Autodesk Fusion 360 part; units mm, degrees
(part 2 of 3)
  line L639 (-140.3467, 118.52) -> (-149.3467, 118.52)
  line L640 (-149.3467, 118.52) -> (-149.3467, 112.02)
  line L641 (-140.3467, 112.02) -> (-140.3467, 118.52)
  line L642 (-149.3467, 112.02) -> (-140.3467, 112.02)
  line L643 (-148.7467, 117.92) -> (-148.7467, 112.62)
  line L644 (-140.9467, 117.92) -> (-148.7467, 117.92)
  line L645 (-140.9467, 112.62) -> (-140.9467, 117.92)
  line L646 (-158.6, 112.62) -> (-150.8, 112.62)
  line L647 (-150.2, 118.52) -> (-159.2, 118.52)
  line L648 (-159.2, 118.52) -> (-159.2, 112.02)
  line L649 (-150.2, 112.02) -> (-150.2, 118.52)
  line L650 (-159.2, 112.02) -> (-150.2, 112.02)
  line L651 (-158.6, 117.92) -> (-158.6, 112.62)
  line L652 (-150.8, 117.92) -> (-158.6, 117.92)
  line L653 (-150.8, 112.62) -> (-150.8, 117.92)
  line L654 (-10.8, 102.6) -> (-3, 102.6)
  line L655 (-2.4, 108.5) -> (-11.4, 108.5)
  line L656 (-11.4, 108.5) -> (-11.4, 102)
  line L657 (-2.4, 102) -> (-2.4, 108.5)
  line L658 (-11.4, 102) -> (-2.4, 102)
  line L659 (-10.8, 107.9) -> (-10.8, 102.6)
  line L660 (-3, 107.9) -> (-10.8, 107.9)
  line L661 (-3, 102.6) -> (-3, 107.9)
  line L662 (-20.6533, 102.6) -> (-12.8533, 102.6)
  line L663 (-12.2533, 108.5) -> (-21.2533, 108.5)
  line L664 (-21.2533, 108.5) -> (-21.2533, 102)
  line L665 (-12.2533, 102) -> (-12.2533, 108.5)
  line L666 (-21.2533, 102) -> (-12.2533, 102)
  line L667 (-20.6533, 107.9) -> (-20.6533, 102.6)
  line L668 (-12.8533, 107.9) -> (-20.6533, 107.9)
  line L669 (-12.8533, 102.6) -> (-12.8533, 107.9)
  line L670 (-30.5067, 102.6) -> (-22.7067, 102.6)
  line L671 (-22.1067, 108.5) -> (-31.1067, 108.5)
  line L672 (-31.1067, 108.5) -> (-31.1067, 102)
  line L673 (-22.1067, 102) -> (-22.1067, 108.5)
  line L674 (-31.1067, 102) -> (-22.1067, 102)
  line L675 (-30.5067, 107.9) -> (-30.5067, 102.6)
  line L676 (-22.7067, 107.9) -> (-30.5067, 107.9)
  line L677 (-22.7067, 102.6) -> (-22.7067, 107.9)
  line L678 (-40.36, 102.6) -> (-32.56, 102.6)
  line L679 (-31.96, 108.5) -> (-40.96, 108.5)
  line L680 (-40.96, 108.5) -> (-40.96, 102)
  line L681 (-31.96, 102) -> (-31.96, 108.5)
  line L682 (-40.96, 102) -> (-31.96, 102)
  line L683 (-40.36, 107.9) -> (-40.36, 102.6)
  line L684 (-32.56, 107.9) -> (-40.36, 107.9)
  line L685 (-32.56, 102.6) -> (-32.56, 107.9)
  line L686 (-50.2133, 102.6) -> (-42.4133, 102.6)
  line L687 (-41.8133, 108.5) -> (-50.8133, 108.5)
  line L688 (-50.8133, 108.5) -> (-50.8133, 102)
  line L689 (-41.8133, 102) -> (-41.8133, 108.5)
  line L690 (-50.8133, 102) -> (-41.8133, 102)
  line L691 (-50.2133, 107.9) -> (-50.2133, 102.6)
  line L692 (-42.4133, 107.9) -> (-50.2133, 107.9)
  line L693 (-42.4133, 102.6) -> (-42.4133, 107.9)
  line L694 (-60.0667, 102.6) -> (-52.2667, 102.6)
  line L695 (-51.6667, 108.5) -> (-60.6667, 108.5)
  line L696 (-60.6667, 108.5) -> (-60.6667, 102)
  line L697 (-51.6667, 102) -> (-51.6667, 108.5)
  line L698 (-60.6667, 102) -> (-51.6667, 102)
  line L699 (-60.0667, 107.9) -> (-60.0667, 102.6)
  line L700 (-52.2667, 107.9) -> (-60.0667, 107.9)
  line L701 (-52.2667, 102.6) -> (-52.2667, 107.9)
  line L702 (-69.92, 102.6) -> (-62.12, 102.6)
  line L703 (-61.52, 108.5) -> (-70.52, 108.5)
  line L704 (-70.52, 108.5) -> (-70.52, 102)
  line L705 (-61.52, 102) -> (-61.52, 108.5)
  line L706 (-70.52, 102) -> (-61.52, 102)
  line L707 (-69.92, 107.9) -> (-69.92, 102.6)
  line L708 (-62.12, 107.9) -> (-69.92, 107.9)
  line L709 (-62.12, 102.6) -> (-62.12, 107.9)
  line L710 (-79.7733, 102.6) -> (-71.9733, 102.6)
  line L711 (-71.3733, 108.5) -> (-80.3733, 108.5)
  line L712 (-80.3733, 108.5) -> (-80.3733, 102)
  line L713 (-71.3733, 102) -> (-71.3733, 108.5)
  line L714 (-80.3733, 102) -> (-71.3733, 102)
  line L715 (-79.7733, 107.9) -> (-79.7733, 102.6)
  line L716 (-71.9733, 107.9) -> (-79.7733, 107.9)
  line L717 (-71.9733, 102.6) -> (-71.9733, 107.9)
  line L718 (-89.6267, 102.6) -> (-81.8267, 102.6)
  line L719 (-81.2267, 108.5) -> (-90.2267, 108.5)
  line L720 (-90.2267, 108.5) -> (-90.2267, 102)
  line L721 (-81.2267, 102) -> (-81.2267, 108.5)
  line L722 (-90.2267, 102) -> (-81.2267, 102)
  line L723 (-89.6267, 107.9) -> (-89.6267, 102.6)
  line L724 (-81.8267, 107.9) -> (-89.6267, 107.9)
  line L725 (-81.8267, 102.6) -> (-81.8267, 107.9)
  line L726 (-99.48, 102.6) -> (-91.68, 102.6)
  line L727 (-91.08, 108.5) -> (-100.08, 108.5)
  line L728 (-100.08, 108.5) -> (-100.08, 102)
  line L729 (-91.08, 102) -> (-91.08, 108.5)
  line L730 (-100.08, 102) -> (-91.08, 102)
  line L731 (-99.48, 107.9) -> (-99.48, 102.6)
  line L732 (-91.68, 107.9) -> (-99.48, 107.9)
  line L733 (-91.68, 102.6) -> (-91.68, 107.9)
  line L734 (-109.3333, 102.6) -> (-101.5333, 102.6)
  line L735 (-100.9333, 108.5) -> (-109.9333, 108.5)
  line L736 (-109.9333, 108.5) -> (-109.9333, 102)
  line L737 (-100.9333, 102) -> (-100.9333, 108.5)
  line L738 (-109.9333, 102) -> (-100.9333, 102)
  line L739 (-109.3333, 107.9) -> (-109.3333, 102.6)
  line L740 (-101.5333, 107.9) -> (-109.3333, 107.9)
  line L741 (-101.5333, 102.6) -> (-101.5333, 107.9)
  line L742 (-119.1867, 102.6) -> (-111.3867, 102.6)
  line L743 (-110.7867, 108.5) -> (-119.7867, 108.5)
  line L744 (-119.7867, 108.5) -> (-119.7867, 102)
  line L745 (-110.7867, 102) -> (-110.7867, 108.5)
  line L746 (-119.7867, 102) -> (-110.7867, 102)
  line L747 (-119.1867, 107.9) -> (-119.1867, 102.6)
  line L748 (-111.3867, 107.9) -> (-119.1867, 107.9)
  line L749 (-111.3867, 102.6) -> (-111.3867, 107.9)
  line L750 (-129.04, 102.6) -> (-121.24, 102.6)
  line L751 (-120.64, 108.5) -> (-129.64, 108.5)
  line L752 (-129.64, 108.5) -> (-129.64, 102)
  line L753 (-120.64, 102) -> (-120.64, 108.5)
  line L754 (-129.64, 102) -> (-120.64, 102)
  line L755 (-129.04, 107.9) -> (-129.04, 102.6)
  line L756 (-121.24, 107.9) -> (-129.04, 107.9)
  line L757 (-121.24, 102.6) -> (-121.24, 107.9)
  line L758 (-138.8933, 102.6) -> (-131.0933, 102.6)
  line L759 (-130.4933, 108.5) -> (-139.4933, 108.5)
  line L760 (-139.4933, 108.5) -> (-139.4933, 102)
  line L761 (-130.4933, 102) -> (-130.4933, 108.5)
  line L762 (-139.4933, 102) -> (-130.4933, 102)
  line L763 (-138.8933, 107.9) -> (-138.8933, 102.6)
  line L764 (-131.0933, 107.9) -> (-138.8933, 107.9)
  line L765 (-131.0933, 102.6) -> (-131.0933, 107.9)
  line L766 (-148.7467, 102.6) -> (-140.9467, 102.6)
  line L767 (-140.3467, 108.5) -> (-149.3467, 108.5)
  line L768 (-149.3467, 108.5) -> (-149.3467, 102)
  line L769 (-140.3467, 102) -> (-140.3467, 108.5)
  line L770 (-149.3467, 102) -> (-140.3467, 102)
  line L771 (-148.7467, 107.9) -> (-148.7467, 102.6)
  line L772 (-140.9467, 107.9) -> (-148.7467, 107.9)
  line L773 (-140.9467, 102.6) -> (-140.9467, 107.9)
  line L774 (-158.6, 102.6) -> (-150.8, 102.6)
  line L775 (-150.2, 108.5) -> (-159.2, 108.5)
  line L776 (-159.2, 108.5) -> (-159.2, 102)
  line L777 (-150.2, 102) -> (-150.2, 108.5)
  line L778 (-159.2, 102) -> (-150.2, 102)
  line L779 (-158.6, 107.9) -> (-158.6, 102.6)
  line L780 (-150.8, 107.9) -> (-158.6, 107.9)
  line L781 (-150.8, 102.6) -> (-150.8, 107.9)
  line L782 (-10.8, 92.58) -> (-3, 92.58)
  line L783 (-2.4, 98.48) -> (-11.4, 98.48)
  line L784 (-11.4, 98.48) -> (-11.4, 91.98)
  line L785 (-2.4, 91.98) -> (-2.4, 98.48)
  line L786 (-11.4, 91.98) -> (-2.4, 91.98)
  line L787 (-10.8, 97.88) -> (-10.8, 92.58)
  line L788 (-3, 97.88) -> (-10.8, 97.88)
  line L789 (-3, 92.58) -> (-3, 97.88)
  line L790 (-20.6533, 92.58) -> (-12.8533, 92.58)
  line L791 (-12.2533, 98.48) -> (-21.2533, 98.48)
  line L792 (-21.2533, 98.48) -> (-21.2533, 91.98)
  line L793 (-12.2533, 91.98) -> (-12.2533, 98.48)
  line L794 (-21.2533, 91.98) -> (-12.2533, 91.98)
  line L795 (-20.6533, 97.88) -> (-20.6533, 92.58)
  line L796 (-12.8533, 97.88) -> (-20.6533, 97.88)
  line L797 (-12.8533, 92.58) -> (-12.8533, 97.88)
  line L798 (-30.5067, 92.58) -> (-22.7067, 92.58)
  line L799 (-22.1067, 98.48) -> (-31.1067, 98.48)
  line L800 (-31.1067, 98.48) -> (-31.1067, 91.98)
  line L801 (-22.1067, 91.98) -> (-22.1067, 98.48)
  line L802 (-31.1067, 91.98) -> (-22.1067, 91.98)
  line L803 (-30.5067, 97.88) -> (-30.5067, 92.58)
  line L804 (-22.7067, 97.88) -> (-30.5067, 97.88)
  line L805 (-22.7067, 92.58) -> (-22.7067, 97.88)
  line L806 (-40.36, 92.58) -> (-32.56, 92.58)
  line L807 (-31.96, 98.48) -> (-40.96, 98.48)
  line L808 (-40.96, 98.48) -> (-40.96, 91.98)
  line L809 (-31.96, 91.98) -> (-31.96, 98.48)
  line L810 (-40.96, 91.98) -> (-31.96, 91.98)
  line L811 (-40.36, 97.88) -> (-40.36, 92.58)
  line L812 (-32.56, 97.88) -> (-40.36, 97.88)
  line L813 (-32.56, 92.58) -> (-32.56, 97.88)
  line L814 (-50.2133, 92.58) -> (-42.4133, 92.58)
  line L815 (-41.8133, 98.48) -> (-50.8133, 98.48)
  line L816 (-50.8133, 98.48) -> (-50.8133, 91.98)
  line L817 (-41.8133, 91.98) -> (-41.8133, 98.48)
  line L818 (-50.8133, 91.98) -> (-41.8133, 91.98)
  line L819 (-50.2133, 97.88) -> (-50.2133, 92.58)
  line L820 (-42.4133, 97.88) -> (-50.2133, 97.88)
  line L821 (-42.4133, 92.58) -> (-42.4133, 97.88)
  line L822 (-60.0667, 92.58) -> (-52.2667, 92.58)
  line L823 (-51.6667, 98.48) -> (-60.6667, 98.48)
  line L824 (-60.6667, 98.48) -> (-60.6667, 91.98)
  line L825 (-51.6667, 91.98) -> (-51.6667, 98.48)
  line L826 (-60.6667, 91.98) -> (-51.6667, 91.98)
  line L827 (-60.0667, 97.88) -> (-60.0667, 92.58)
  line L828 (-52.2667, 97.88) -> (-60.0667, 97.88)
  line L829 (-52.2667, 92.58) -> (-52.2667, 97.88)
  line L830 (-69.92, 92.58) -> (-62.12, 92.58)
  line L831 (-61.52, 98.48) -> (-70.52, 98.48)
  line L832 (-70.52, 98.48) -> (-70.52, 91.98)
  line L833 (-61.52, 91.98) -> (-61.52, 98.48)
  line L834 (-70.52, 91.98) -> (-61.52, 91.98)
  line L835 (-69.92, 97.88) -> (-69.92, 92.58)
  line L836 (-62.12, 97.88) -> (-69.92, 97.88)
  line L837 (-62.12, 92.58) -> (-62.12, 97.88)
  line L838 (-79.7733, 92.58) -> (-71.9733, 92.58)
  line L839 (-71.3733, 98.48) -> (-80.3733, 98.48)
  line L840 (-80.3733, 98.48) -> (-80.3733, 91.98)
  line L841 (-71.3733, 91.98) -> (-71.3733, 98.48)
  line L842 (-80.3733, 91.98) -> (-71.3733, 91.98)
  line L843 (-79.7733, 97.88) -> (-79.7733, 92.58)
  line L844 (-71.9733, 97.88) -> (-79.7733, 97.88)
  line L845 (-71.9733, 92.58) -> (-71.9733, 97.88)
  line L846 (-89.6267, 92.58) -> (-81.8267, 92.58)
  line L847 (-81.2267, 98.48) -> (-90.2267, 98.48)
  line L848 (-90.2267, 98.48) -> (-90.2267, 91.98)
  line L849 (-81.2267, 91.98) -> (-81.2267, 98.48)
  line L850 (-90.2267, 91.98) -> (-81.2267, 91.98)
  line L851 (-89.6267, 97.88) -> (-89.6267, 92.58)
  line L852 (-81.8267, 97.88) -> (-89.6267, 97.88)
  line L853 (-81.8267, 92.58) -> (-81.8267, 97.88)
  line L854 (-99.48, 92.58) -> (-91.68, 92.58)
  line L855 (-91.08, 98.48) -> (-100.08, 98.48)
  line L856 (-100.08, 98.48) -> (-100.08, 91.98)
  line L857 (-91.08, 91.98) -> (-91.08, 98.48)
  line L858 (-100.08, 91.98) -> (-91.08, 91.98)
  line L859 (-99.48, 97.88) -> (-99.48, 92.58)
  line L860 (-91.68, 97.88) -> (-99.48, 97.88)
  line L861 (-91.68, 92.58) -> (-91.68, 97.88)
  line L862 (-109.3333, 92.58) -> (-101.5333, 92.58)
  line L863 (-100.9333, 98.48) -> (-109.9333, 98.48)
  line L864 (-109.9333, 98.48) -> (-109.9333, 91.98)
  line L865 (-100.9333, 91.98) -> (-100.9333, 98.48)
  line L866 (-109.9333, 91.98) -> (-100.9333, 91.98)
  line L867 (-109.3333, 97.88) -> (-109.3333, 92.58)
  line L868 (-101.5333, 97.88) -> (-109.3333, 97.88)
  line L869 (-101.5333, 92.58) -> (-101.5333, 97.88)
  line L870 (-119.1867, 92.58) -> (-111.3867, 92.58)
  line L871 (-110.7867, 98.48) -> (-119.7867, 98.48)
  line L872 (-119.7867, 98.48) -> (-119.7867, 91.98)
  line L873 (-110.7867, 91.98) -> (-110.7867, 98.48)
  line L874 (-119.7867, 91.98) -> (-110.7867, 91.98)
  line L875 (-119.1867, 97.88) -> (-119.1867, 92.58)
  line L876 (-111.3867, 97.88) -> (-119.1867, 97.88)
  line L877 (-111.3867, 92.58) -> (-111.3867, 97.88)
  line L878 (-129.04, 92.58) -> (-121.24, 92.58)
  line L879 (-120.64, 98.48) -> (-129.64, 98.48)
  line L880 (-129.64, 98.48) -> (-129.64, 91.98)
  line L881 (-120.64, 91.98) -> (-120.64, 98.48)
  line L882 (-129.64, 91.98) -> (-120.64, 91.98)
  line L883 (-129.04, 97.88) -> (-129.04, 92.58)
  line L884 (-121.24, 97.88) -> (-129.04, 97.88)
  line L885 (-121.24, 92.58) -> (-121.24, 97.88)
  line L886 (-138.8933, 92.58) -> (-131.0933, 92.58)
  line L887 (-130.4933, 98.48) -> (-139.4933, 98.48)
  line L888 (-139.4933, 98.48) -> (-139.4933, 91.98)
  line L889 (-130.4933, 91.98) -> (-130.4933, 98.48)
  line L890 (-139.4933, 91.98) -> (-130.4933, 91.98)
  line L891 (-138.8933, 97.88) -> (-138.8933, 92.58)
  line L892 (-131.0933, 97.88) -> (-138.8933, 97.88)
  line L893 (-131.0933, 92.58) -> (-131.0933, 97.88)
  line L894 (-148.7467, 92.58) -> (-140.9467, 92.58)
  line L895 (-140.3467, 98.48) -> (-149.3467, 98.48)
  line L896 (-149.3467, 98.48) -> (-149.3467, 91.98)
  line L897 (-140.3467, 91.98) -> (-140.3467, 98.48)
  line L898 (-149.3467, 91.98) -> (-140.3467, 91.98)
  line L899 (-148.7467, 97.88) -> (-148.7467, 92.58)
  line L900 (-140.9467, 97.88) -> (-148.7467, 97.88)
  line L901 (-140.9467, 92.58) -> (-140.9467, 97.88)
  line L902 (-158.6, 92.58) -> (-150.8, 92.58)
  line L903 (-150.2, 98.48) -> (-159.2, 98.48)
  line L904 (-159.2, 98.48) -> (-159.2, 91.98)
  line L905 (-150.2, 91.98) -> (-150.2, 98.48)
  line L906 (-159.2, 91.98) -> (-150.2, 91.98)
  line L907 (-158.6, 97.88) -> (-158.6, 92.58)
  line L908 (-150.8, 97.88) -> (-158.6, 97.88)
  line L909 (-150.8, 92.58) -> (-150.8, 97.88)
  line L910 (-10.8, 82.56) -> (-3, 82.56)
  line L911 (-2.4, 88.46) -> (-11.4, 88.46)
  line L912 (-11.4, 88.46) -> (-11.4, 81.96)
  line L913 (-2.4, 81.96) -> (-2.4, 88.46)
  line L914 (-11.4, 81.96) -> (-2.4, 81.96)
  line L915 (-10.8, 87.86) -> (-10.8, 82.56)
  line L916 (-3, 87.86) -> (-10.8, 87.86)
  line L917 (-3, 82.56) -> (-3, 87.86)
  line L918 (-20.6533, 82.56) -> (-12.8533, 82.56)
  line L919 (-12.2533, 88.46) -> (-21.2533, 88.46)
  line L920 (-21.2533, 88.46) -> (-21.2533, 81.96)
  line L921 (-12.2533, 81.96) -> (-12.2533, 88.46)
  line L922 (-21.2533, 81.96) -> (-12.2533, 81.96)
  line L923 (-20.6533, 87.86) -> (-20.6533, 82.56)
  line L924 (-12.8533, 87.86) -> (-20.6533, 87.86)
  line L925 (-12.8533, 82.56) -> (-12.8533, 87.86)
  line L926 (-30.5067, 82.56) -> (-22.7067, 82.56)
  line L927 (-22.1067, 88.46) -> (-31.1067, 88.46)
  line L928 (-31.1067, 88.46) -> (-31.1067, 81.96)
  line L929 (-22.1067, 81.96) -> (-22.1067, 88.46)
  line L930 (-31.1067, 81.96) -> (-22.1067, 81.96)
  line L931 (-30.5067, 87.86) -> (-30.5067, 82.56)
  line L932 (-22.7067, 87.86) -> (-30.5067, 87.86)
  line L933 (-22.7067, 82.56) -> (-22.7067, 87.86)
  line L934 (-40.36, 82.56) -> (-32.56, 82.56)
  line L935 (-31.96, 88.46) -> (-40.96, 88.46)
  line L936 (-40.96, 88.46) -> (-40.96, 81.96)
  line L937 (-31.96, 81.96) -> (-31.96, 88.46)
  line L938 (-40.96, 81.96) -> (-31.96, 81.96)
  line L939 (-40.36, 87.86) -> (-40.36, 82.56)
  line L940 (-32.56, 87.86) -> (-40.36, 87.86)
  line L941 (-32.56, 82.56) -> (-32.56, 87.86)
  line L942 (-50.2133, 82.56) -> (-42.4133, 82.56)
  line L943 (-41.8133, 88.46) -> (-50.8133, 88.46)
  line L944 (-50.8133, 88.46) -> (-50.8133, 81.96)
  line L945 (-41.8133, 81.96) -> (-41.8133, 88.46)
  line L946 (-50.8133, 81.96) -> (-41.8133, 81.96)
  line L947 (-50.2133, 87.86) -> (-50.2133, 82.56)
  line L948 (-42.4133, 87.86) -> (-50.2133, 87.86)
  line L949 (-42.4133, 82.56) -> (-42.4133, 87.86)
  line L950 (-60.0667, 82.56) -> (-52.2667, 82.56)
  line L951 (-51.6667, 88.46) -> (-60.6667, 88.46)
  line L952 (-60.6667, 88.46) -> (-60.6667, 81.96)
  line L953 (-51.6667, 81.96) -> (-51.6667, 88.46)
  line L954 (-60.6667, 81.96) -> (-51.6667, 81.96)
  line L955 (-60.0667, 87.86) -> (-60.0667, 82.56)
  line L956 (-52.2667, 87.86) -> (-60.0667, 87.86)
  line L957 (-52.2667, 82.56) -> (-52.2667, 87.86)
  line L958 (-69.92, 82.56) -> (-62.12, 82.56)
  line L959 (-61.52, 88.46) -> (-70.52, 88.46)
  line L960 (-70.52, 88.46) -> (-70.52, 81.96)
  line L961 (-61.52, 81.96) -> (-61.52, 88.46)
  line L962 (-70.52, 81.96) -> (-61.52, 81.96)
  line L963 (-69.92, 87.86) -> (-69.92, 82.56)
  line L964 (-62.12, 87.86) -> (-69.92, 87.86)
  line L965 (-62.12, 82.56) -> (-62.12, 87.86)
  line L966 (-79.7733, 82.56) -> (-71.9733, 82.56)
  line L967 (-71.3733, 88.46) -> (-80.3733, 88.46)
  line L968 (-80.3733, 88.46) -> (-80.3733, 81.96)
  line L969 (-71.3733, 81.96) -> (-71.3733, 88.46)
  line L970 (-80.3733, 81.96) -> (-71.3733, 81.96)
  line L971 (-79.7733, 87.86) -> (-79.7733, 82.56)
  line L972 (-71.9733, 87.86) -> (-79.7733, 87.86)
  line L973 (-71.9733, 82.56) -> (-71.9733, 87.86)
  line L974 (-89.6267, 82.56) -> (-81.8267, 82.56)
  line L975 (-81.2267, 88.46) -> (-90.2267, 88.46)
  line L976 (-90.2267, 88.46) -> (-90.2267, 81.96)
  line L977 (-81.2267, 81.96) -> (-81.2267, 88.46)
  line L978 (-90.2267, 81.96) -> (-81.2267, 81.96)
  line L979 (-89.6267, 87.86) -> (-89.6267, 82.56)
  line L980 (-81.8267, 87.86) -> (-89.6267, 87.86)
  line L981 (-81.8267, 82.56) -> (-81.8267, 87.86)
  line L982 (-99.48, 82.56) -> (-91.68, 82.56)
  line L983 (-91.08, 88.46) -> (-100.08, 88.46)
  line L984 (-100.08, 88.46) -> (-100.08, 81.96)
  line L985 (-91.08, 81.96) -> (-91.08, 88.46)
  line L986 (-100.08, 81.96) -> (-91.08, 81.96)
  line L987 (-99.48, 87.86) -> (-99.48, 82.56)
  line L988 (-91.68, 87.86) -> (-99.48, 87.86)
  line L989 (-91.68, 82.56) -> (-91.68, 87.86)
  line L990 (-109.3333, 82.56) -> (-101.5333, 82.56)
  line L991 (-100.9333, 88.46) -> (-109.9333, 88.46)
  line L992 (-109.9333, 88.46) -> (-109.9333, 81.96)
  line L993 (-100.9333, 81.96) -> (-100.9333, 88.46)
  line L994 (-109.9333, 81.96) -> (-100.9333, 81.96)
  line L995 (-109.3333, 87.86) -> (-109.3333, 82.56)
  line L996 (-101.5333, 87.86) -> (-109.3333, 87.86)
  line L997 (-101.5333, 82.56) -> (-101.5333, 87.86)
  line L998 (-119.1867, 82.56) -> (-111.3867, 82.56)
  line L999 (-110.7867, 88.46) -> (-119.7867, 88.46)
  line L1000 (-119.7867, 88.46) -> (-119.7867, 81.96)
  line L1001 (-110.7867, 81.96) -> (-110.7867, 88.46)
  line L1002 (-119.7867, 81.96) -> (-110.7867, 81.96)
  line L1003 (-119.1867, 87.86) -> (-119.1867, 82.56)
  line L1004 (-111.3867, 87.86) -> (-119.1867, 87.86)
  line L1005 (-111.3867, 82.56) -> (-111.3867, 87.86)
  line L1006 (-129.04, 82.56) -> (-121.24, 82.56)
  line L1007 (-120.64, 88.46) -> (-129.64, 88.46)
  line L1008 (-129.64, 88.46) -> (-129.64, 81.96)
  line L1009 (-120.64, 81.96) -> (-120.64, 88.46)
  line L1010 (-129.64, 81.96) -> (-120.64, 81.96)
  line L1011 (-129.04, 87.86) -> (-129.04, 82.56)
  line L1012 (-121.24, 87.86) -> (-129.04, 87.86)
  line L1013 (-121.24, 82.56) -> (-121.24, 87.86)
  line L1014 (-138.8933, 82.56) -> (-131.0933, 82.56)
  line L1015 (-130.4933, 88.46) -> (-139.4933, 88.46)
  line L1016 (-139.4933, 88.46) -> (-139.4933, 81.96)
  line L1017 (-130.4933, 81.96) -> (-130.4933, 88.46)
  line L1018 (-139.4933, 81.96) -> (-130.4933, 81.96)
  line L1019 (-138.8933, 87.86) -> (-138.8933, 82.56)
  line L1020 (-131.0933, 87.86) -> (-138.8933, 87.86)
  line L1021 (-131.0933, 82.56) -> (-131.0933, 87.86)
  line L1022 (-148.7467, 82.56) -> (-140.9467, 82.56)
  line L1023 (-140.3467, 88.46) -> (-149.3467, 88.46)
  line L1024 (-149.3467, 88.46) -> (-149.3467, 81.96)
  line L1025 (-140.3467, 81.96) -> (-140.3467, 88.46)
  line L1026 (-149.3467, 81.96) -> (-140.3467, 81.96)
  line L1027 (-148.7467, 87.86) -> (-148.7467, 82.56)
  line L1028 (-140.9467, 87.86) -> (-148.7467, 87.86)
  line L1029 (-140.9467, 82.56) -> (-140.9467, 87.86)
  line L1030 (-158.6, 82.56) -> (-150.8, 82.56)
  line L1031 (-150.2, 88.46) -> (-159.2, 88.46)
  line L1032 (-159.2, 88.46) -> (-159.2, 81.96)
  line L1033 (-150.2, 81.96) -> (-150.2, 88.46)
  line L1034 (-159.2, 81.96) -> (-150.2, 81.96)
  line L1035 (-158.6, 87.86) -> (-158.6, 82.56)
  line L1036 (-150.8, 87.86) -> (-158.6, 87.86)
  line L1037 (-150.8, 82.56) -> (-150.8, 87.86)
  line L1038 (-10.8, 72.54) -> (-3, 72.54)
  line L1039 (-2.4, 78.44) -> (-11.4, 78.44)
  line L1040 (-11.4, 78.44) -> (-11.4, 71.94)
  line L1041 (-2.4, 71.94) -> (-2.4, 78.44)
  line L1042 (-11.4, 71.94) -> (-2.4, 71.94)
  line L1043 (-10.8, 77.84) -> (-10.8, 72.54)
  line L1044 (-3, 77.84) -> (-10.8, 77.84)
  line L1045 (-3, 72.54) -> (-3, 77.84)
  line L1046 (-20.6533, 72.54) -> (-12.8533, 72.54)
  line L1047 (-12.2533, 78.44) -> (-21.2533, 78.44)
  line L1048 (-21.2533, 78.44) -> (-21.2533, 71.94)
  line L1049 (-12.2533, 71.94) -> (-12.2533, 78.44)
  line L1050 (-21.2533, 71.94) -> (-12.2533, 71.94)
  line L1051 (-20.6533, 77.84) -> (-20.6533, 72.54)
  line L1052 (-12.8533, 77.84) -> (-20.6533, 77.84)
  line L1053 (-12.8533, 72.54) -> (-12.8533, 77.84)
  line L1054 (-30.5067, 72.54) -> (-22.7067, 72.54)
  line L1055 (-22.1067, 78.44) -> (-31.1067, 78.44)
  line L1056 (-31.1067, 78.44) -> (-31.1067, 71.94)
  line L1057 (-22.1067, 71.94) -> (-22.1067, 78.44)
  line L1058 (-31.1067, 71.94) -> (-22.1067, 71.94)
  line L1059 (-30.5067, 77.84) -> (-30.5067, 72.54)
  line L1060 (-22.7067, 77.84) -> (-30.5067, 77.84)
  line L1061 (-22.7067, 72.54) -> (-22.7067, 77.84)
  line L1062 (-40.36, 72.54) -> (-32.56, 72.54)
  line L1063 (-31.96, 78.44) -> (-40.96, 78.44)
  line L1064 (-40.96, 78.44) -> (-40.96, 71.94)
  line L1065 (-31.96, 71.94) -> (-31.96, 78.44)
  line L1066 (-40.96, 71.94) -> (-31.96, 71.94)
  line L1067 (-40.36, 77.84) -> (-40.36, 72.54)
  line L1068 (-32.56, 77.84) -> (-40.36, 77.84)
  line L1069 (-32.56, 72.54) -> (-32.56, 77.84)
  line L1070 (-50.2133, 72.54) -> (-42.4133, 72.54)
  line L1071 (-41.8133, 78.44) -> (-50.8133, 78.44)
  line L1072 (-50.8133, 78.44) -> (-50.8133, 71.94)
  line L1073 (-41.8133, 71.94) -> (-41.8133, 78.44)
  line L1074 (-50.8133, 71.94) -> (-41.8133, 71.94)
  line L1075 (-50.2133, 77.84) -> (-50.2133, 72.54)
  line L1076 (-42.4133, 77.84) -> (-50.2133, 77.84)
  line L1077 (-42.4133, 72.54) -> (-42.4133, 77.84)
  line L1078 (-60.0667, 72.54) -> (-52.2667, 72.54)
  line L1079 (-51.6667, 78.44) -> (-60.6667, 78.44)
  line L1080 (-60.6667, 78.44) -> (-60.6667, 71.94)
  line L1081 (-51.6667, 71.94) -> (-51.6667, 78.44)
  line L1082 (-60.6667, 71.94) -> (-51.6667, 71.94)
  line L1083 (-60.0667, 77.84) -> (-60.0667, 72.54)
  line L1084 (-52.2667, 77.84) -> (-60.0667, 77.84)
  line L1085 (-52.2667, 72.54) -> (-52.2667, 77.84)
  line L1086 (-69.92, 72.54) -> (-62.12, 72.54)
  line L1087 (-61.52, 78.44) -> (-70.52, 78.44)
  line L1088 (-70.52, 78.44) -> (-70.52, 71.94)
  line L1089 (-61.52, 71.94) -> (-61.52, 78.44)
  line L1090 (-70.52, 71.94) -> (-61.52, 71.94)
  line L1091 (-69.92, 77.84) -> (-69.92, 72.54)
  line L1092 (-62.12, 77.84) -> (-69.92, 77.84)
  line L1093 (-62.12, 72.54) -> (-62.12, 77.84)
  line L1094 (-79.7733, 72.54) -> (-71.9733, 72.54)
  line L1095 (-71.3733, 78.44) -> (-80.3733, 78.44)
  line L1096 (-80.3733, 78.44) -> (-80.3733, 71.94)
  line L1097 (-71.3733, 71.94) -> (-71.3733, 78.44)
  line L1098 (-80.3733, 71.94) -> (-71.3733, 71.94)
  line L1099 (-79.7733, 77.84) -> (-79.7733, 72.54)
  line L1100 (-71.9733, 77.84) -> (-79.7733, 77.84)
  line L1101 (-71.9733, 72.54) -> (-71.9733, 77.84)
  line L1102 (-89.6267, 72.54) -> (-81.8267, 72.54)
  line L1103 (-81.2267, 78.44) -> (-90.2267, 78.44)
  line L1104 (-90.2267, 78.44) -> (-90.2267, 71.94)
  line L1105 (-81.2267, 71.94) -> (-81.2267, 78.44)
  line L1106 (-90.2267, 71.94) -> (-81.2267, 71.94)
  line L1107 (-89.6267, 77.84) -> (-89.6267, 72.54)
  line L1108 (-81.8267, 77.84) -> (-89.6267, 77.84)
  line L1109 (-81.8267, 72.54) -> (-81.8267, 77.84)
  line L1110 (-99.48, 72.54) -> (-91.68, 72.54)
  line L1111 (-91.08, 78.44) -> (-100.08, 78.44)
  line L1112 (-100.08, 78.44) -> (-100.08, 71.94)
  line L1113 (-91.08, 71.94) -> (-91.08, 78.44)
  line L1114 (-100.08, 71.94) -> (-91.08, 71.94)
  line L1115 (-99.48, 77.84) -> (-99.48, 72.54)
  line L1116 (-91.68, 77.84) -> (-99.48, 77.84)
  line L1117 (-91.68, 72.54) -> (-91.68, 77.84)
  line L1118 (-109.3333, 72.54) -> (-101.5333, 72.54)
  line L1119 (-100.9333, 78.44) -> (-109.9333, 78.44)
  line L1120 (-109.9333, 78.44) -> (-109.9333, 71.94)
  line L1121 (-100.9333, 71.94) -> (-100.9333, 78.44)
  line L1122 (-109.9333, 71.94) -> (-100.9333, 71.94)
  line L1123 (-109.3333, 77.84) -> (-109.3333, 72.54)
  line L1124 (-101.5333, 77.84) -> (-109.3333, 77.84)
  line L1125 (-101.5333, 72.54) -> (-101.5333, 77.84)
  line L1126 (-119.1867, 72.54) -> (-111.3867, 72.54)
  line L1127 (-110.7867, 78.44) -> (-119.7867, 78.44)
  line L1128 (-119.7867, 78.44) -> (-119.7867, 71.94)
  line L1129 (-110.7867, 71.94) -> (-110.7867, 78.44)
  line L1130 (-119.7867, 71.94) -> (-110.7867, 71.94)
  line L1131 (-119.1867, 77.84) -> (-119.1867, 72.54)
  line L1132 (-111.3867, 77.84) -> (-119.1867, 77.84)
  line L1133 (-111.3867, 72.54) -> (-111.3867, 77.84)
  line L1134 (-129.04, 72.54) -> (-121.24, 72.54)
  line L1135 (-120.64, 78.44) -> (-129.64, 78.44)
  line L1136 (-129.64, 78.44) -> (-129.64, 71.94)
  line L1137 (-120.64, 71.94) -> (-120.64, 78.44)
  line L1138 (-129.64, 71.94) -> (-120.64, 71.94)
  line L1139 (-129.04, 77.84) -> (-129.04, 72.54)
  line L1140 (-121.24, 77.84) -> (-129.04, 77.84)
  line L1141 (-121.24, 72.54) -> (-121.24, 77.84)
  line L1142 (-138.8933, 72.54) -> (-131.0933, 72.54)
  line L1143 (-130.4933, 78.44) -> (-139.4933, 78.44)
  line L1144 (-139.4933, 78.44) -> (-139.4933, 71.94)
  line L1145 (-130.4933, 71.94) -> (-130.4933, 78.44)
  line L1146 (-139.4933, 71.94) -> (-130.4933, 71.94)
  line L1147 (-138.8933, 77.84) -> (-138.8933, 72.54)
  line L1148 (-131.0933, 77.84) -> (-138.8933, 77.84)
  line L1149 (-131.0933, 72.54) -> (-131.0933, 77.84)
  line L1150 (-148.7467, 72.54) -> (-140.9467, 72.54)
  line L1151 (-140.3467, 78.44) -> (-149.3467, 78.44)
  line L1152 (-149.3467, 78.44) -> (-149.3467, 71.94)
  line L1153 (-140.3467, 71.94) -> (-140.3467, 78.44)
  line L1154 (-149.3467, 71.94) -> (-140.3467, 71.94)
  line L1155 (-148.7467, 77.84) -> (-148.7467, 72.54)
  line L1156 (-140.9467, 77.84) -> (-148.7467, 77.84)
  line L1157 (-140.9467, 72.54) -> (-140.9467, 77.84)
  line L1158 (-158.6, 72.54) -> (-150.8, 72.54)
  line L1159 (-150.2, 78.44) -> (-159.2, 78.44)
  line L1160 (-159.2, 78.44) -> (-159.2, 71.94)
  line L1161 (-150.2, 71.94) -> (-150.2, 78.44)
  line L1162 (-159.2, 71.94) -> (-150.2, 71.94)
  line L1163 (-158.6, 77.84) -> (-158.6, 72.54)
  line L1164 (-150.8, 77.84) -> (-158.6, 77.84)
  line L1165 (-150.8, 72.54) -> (-150.8, 77.84)
  line L1166 (-10.8, 62.52) -> (-3, 62.52)
  line L1167 (-2.4, 68.42) -> (-11.4, 68.42)
  line L1168 (-11.4, 68.42) -> (-11.4, 61.92)
  line L1169 (-2.4, 61.92) -> (-2.4, 68.42)
  line L1170 (-11.4, 61.92) -> (-2.4, 61.92)
  line L1171 (-10.8, 67.82) -> (-10.8, 62.52)
  line L1172 (-3, 67.82) -> (-10.8, 67.82)
  line L1173 (-3, 62.52) -> (-3, 67.82)
  line L1174 (-20.6533, 62.52) -> (-12.8533, 62.52)
  line L1175 (-12.2533, 68.42) -> (-21.2533, 68.42)
  line L1176 (-21.2533, 68.42) -> (-21.2533, 61.92)
  line L1177 (-12.2533, 61.92) -> (-12.2533, 68.42)
  line L1178 (-21.2533, 61.92) -> (-12.2533, 61.92)
  line L1179 (-20.6533, 67.82) -> (-20.6533, 62.52)
  line L1180 (-12.8533, 67.82) -> (-20.6533, 67.82)
  line L1181 (-12.8533, 62.52) -> (-12.8533, 67.82)
  line L1182 (-30.5067, 62.52) -> (-22.7067, 62.52)
  line L1183 (-22.1067, 68.42) -> (-31.1067, 68.42)
  line L1184 (-31.1067, 68.42) -> (-31.1067, 61.92)
  line L1185 (-22.1067, 61.92) -> (-22.1067, 68.42)
  line L1186 (-31.1067, 61.92) -> (-22.1067, 61.92)
  line L1187 (-30.5067, 67.82) -> (-30.5067, 62.52)
  line L1188 (-22.7067, 67.82) -> (-30.5067, 67.82)
  line L1189 (-22.7067, 62.52) -> (-22.7067, 67.82)
  line L1190 (-40.36, 62.52) -> (-32.56, 62.52)
  line L1191 (-31.96, 68.42) -> (-40.96, 68.42)
  line L1192 (-40.96, 68.42) -> (-40.96, 61.92)
  line L1193 (-31.96, 61.92) -> (-31.96, 68.42)
  line L1194 (-40.96, 61.92) -> (-31.96, 61.92)
  line L1195 (-40.36, 67.82) -> (-40.36, 62.52)
  line L1196 (-32.56, 67.82) -> (-40.36, 67.82)
  line L1197 (-32.56, 62.52) -> (-32.56, 67.82)
  line L1198 (-50.2133, 62.52) -> (-42.4133, 62.52)
  line L1199 (-41.8133, 68.42) -> (-50.8133, 68.42)
  line L1200 (-50.8133, 68.42) -> (-50.8133, 61.92)
  line L1201 (-41.8133, 61.92) -> (-41.8133, 68.42)
  line L1202 (-50.8133, 61.92) -> (-41.8133, 61.92)
  line L1203 (-50.2133, 67.82) -> (-50.2133, 62.52)
  line L1204 (-42.4133, 67.82) -> (-50.2133, 67.82)
  line L1205 (-42.4133, 62.52) -> (-42.4133, 67.82)
  line L1206 (-60.0667, 62.52) -> (-52.2667, 62.52)
  line L1207 (-51.6667, 68.42) -> (-60.6667, 68.42)
  line L1208 (-60.6667, 68.42) -> (-60.6667, 61.92)
  line L1209 (-51.6667, 61.92) -> (-51.6667, 68.42)
  line L1210 (-60.6667, 61.92) -> (-51.6667, 61.92)
  line L1211 (-60.0667, 67.82) -> (-60.0667, 62.52)
  line L1212 (-52.2667, 67.82) -> (-60.0667, 67.82)
  line L1213 (-52.2667, 62.52) -> (-52.2667, 67.82)
  line L1214 (-69.92, 62.52) -> (-62.12, 62.52)
  line L1215 (-61.52, 68.42) -> (-70.52, 68.42)
  line L1216 (-70.52, 68.42) -> (-70.52, 61.92)
  line L1217 (-61.52, 61.92) -> (-61.52, 68.42)
  line L1218 (-70.52, 61.92) -> (-61.52, 61.92)
  line L1219 (-69.92, 67.82) -> (-69.92, 62.52)
  line L1220 (-62.12, 67.82) -> (-69.92, 67.82)
  line L1221 (-62.12, 62.52) -> (-62.12, 67.82)
  line L1222 (-79.7733, 62.52) -> (-71.9733, 62.52)
  line L1223 (-71.3733, 68.42) -> (-80.3733, 68.42)
  line L1224 (-80.3733, 68.42) -> (-80.3733, 61.92)
  line L1225 (-71.3733, 61.92) -> (-71.3733, 68.42)
  line L1226 (-80.3733, 61.92) -> (-71.3733, 61.92)
  line L1227 (-79.7733, 67.82) -> (-79.7733, 62.52)
  line L1228 (-71.9733, 67.82) -> (-79.7733, 67.82)
  line L1229 (-71.9733, 62.52) -> (-71.9733, 67.82)
  line L1230 (-89.6267, 62.52) -> (-81.8267, 62.52)
  line L1231 (-81.2267, 68.42) -> (-90.2267, 68.42)
  line L1232 (-90.2267, 68.42) -> (-90.2267, 61.92)
  line L1233 (-81.2267, 61.92) -> (-81.2267, 68.42)
  line L1234 (-90.2267, 61.92) -> (-81.2267, 61.92)
  line L1235 (-89.6267, 67.82) -> (-89.6267, 62.52)
  line L1236 (-81.8267, 67.82) -> (-89.6267, 67.82)
  line L1237 (-81.8267, 62.52) -> (-81.8267, 67.82)
  line L1238 (-99.48, 62.52) -> (-91.68, 62.52)
  line L1239 (-91.08, 68.42) -> (-100.08, 68.42)
  line L1240 (-100.08, 68.42) -> (-100.08, 61.92)
  line L1241 (-91.08, 61.92) -> (-91.08, 68.42)
  line L1242 (-100.08, 61.92) -> (-91.08, 61.92)
  line L1243 (-99.48, 67.82) -> (-99.48, 62.52)
  line L1244 (-91.68, 67.82) -> (-99.48, 67.82)
  line L1245 (-91.68, 62.52) -> (-91.68, 67.82)
  line L1246 (-109.3333, 62.52) -> (-101.5333, 62.52)
  line L1247 (-100.9333, 68.42) -> (-109.9333, 68.42)
  line L1248 (-109.9333, 68.42) -> (-109.9333, 61.92)
  line L1249 (-100.9333, 61.92) -> (-100.9333, 68.42)
  line L1250 (-109.9333, 61.92) -> (-100.9333, 61.92)
  line L1251 (-109.3333, 67.82) -> (-109.3333, 62.52)
  line L1252 (-101.5333, 67.82) -> (-109.3333, 67.82)
  line L1253 (-101.5333, 62.52) -> (-101.5333, 67.82)
  line L1254 (-119.1867, 62.52) -> (-111.3867, 62.52)
  line L1255 (-110.7867, 68.42) -> (-119.7867, 68.42)
  line L1256 (-119.7867, 68.42) -> (-119.7867, 61.92)
  line L1257 (-110.7867, 61.92) -> (-110.7867, 68.42)
  line L1258 (-119.7867, 61.92) -> (-110.7867, 61.92)
  line L1259 (-119.1867, 67.82) -> (-119.1867, 62.52)
  line L1260 (-111.3867, 67.82) -> (-119.1867, 67.82)
  line L1261 (-111.3867, 62.52) -> (-111.3867, 67.82)
  line L1262 (-129.04, 62.52) -> (-121.24, 62.52)
  line L1263 (-120.64, 68.42) -> (-129.64, 68.42)
  line L1264 (-129.64, 68.42) -> (-129.64, 61.92)
  line L1265 (-120.64, 61.92) -> (-120.64, 68.42)
  line L1266 (-129.64, 61.92) -> (-120.64, 61.92)
  line L1267 (-129.04, 67.82) -> (-129.04, 62.52)
  line L1268 (-121.24, 67.82) -> (-129.04, 67.82)
  line L1269 (-121.24, 62.52) -> (-121.24, 67.82)
  line L1270 (-138.8933, 62.52) -> (-131.0933, 62.52)
  line L1271 (-130.4933, 68.42) -> (-139.4933, 68.42)
  line L1272 (-139.4933, 68.42) -> (-139.4933, 61.92)
  line L1273 (-130.4933, 61.92) -> (-130.4933, 68.42)
  line L1274 (-139.4933, 61.92) -> (-130.4933, 61.92)
  line L1275 (-138.8933, 67.82) -> (-138.8933, 62.52)
  line L1276 (-131.0933, 67.82) -> (-138.8933, 67.82)
  line L1277 (-131.0933, 62.52) -> (-131.0933, 67.82)
  line L1278 (-148.7467, 62.52) -> (-140.9467, 62.52)
  line L1279 (-140.3467, 68.42) -> (-149.3467, 68.42)
  line L1280 (-149.3467, 68.42) -> (-149.3467, 61.92)
  line L1281 (-140.3467, 61.92) -> (-140.3467, 68.42)
  line L1282 (-149.3467, 61.92) -> (-140.3467, 61.92)
  line L1283 (-148.7467, 67.82) -> (-148.7467, 62.52)
  line L1284 (-140.9467, 67.82) -> (-148.7467, 67.82)
  line L1285 (-140.9467, 62.52) -> (-140.9467, 67.82)
  line L1286 (-158.6, 62.52) -> (-150.8, 62.52)
  line L1287 (-150.2, 68.42) -> (-159.2, 68.42)
  line L1288 (-159.2, 68.42) -> (-159.2, 61.92)
  line L1289 (-150.2, 61.92) -> (-150.2, 68.42)
  line L1290 (-159.2, 61.92) -> (-150.2, 61.92)
  line L1291 (-158.6, 67.82) -> (-158.6, 62.52)
  line L1292 (-150.8, 67.82) -> (-158.6, 67.82)
  line L1293 (-150.8, 62.52) -> (-150.8, 67.82)
  line L1294 (-10.8, 52.5) -> (-3, 52.5)
  line L1295 (-2.4, 58.4) -> (-11.4, 58.4)
  line L1296 (-11.4, 58.4) -> (-11.4, 51.9)
  line L1297 (-2.4, 51.9) -> (-2.4, 58.4)
  line L1298 (-11.4, 51.9) -> (-2.4, 51.9)
  line L1299 (-10.8, 57.8) -> (-10.8, 52.5)
  line L1300 (-3, 57.8) -> (-10.8, 57.8)
  line L1301 (-3, 52.5) -> (-3, 57.8)
  line L1302 (-20.6533, 52.5) -> (-12.8533, 52.5)
  line L1303 (-12.2533, 58.4) -> (-21.2533, 58.4)
  line L1304 (-21.2533, 58.4) -> (-21.2533, 51.9)
  line L1305 (-12.2533, 51.9) -> (-12.2533, 58.4)
  line L1306 (-21.2533, 51.9) -> (-12.2533, 51.9)
  line L1307 (-20.6533, 57.8) -> (-20.6533, 52.5)
  line L1308 (-12.8533, 57.8) -> (-20.6533, 57.8)
  line L1309 (-12.8533, 52.5) -> (-12.8533, 57.8)
  line L1310 (-30.5067, 52.5) -> (-22.7067, 52.5)
  line L1311 (-22.1067, 58.4) -> (-31.1067, 58.4)
  line L1312 (-31.1067, 58.4) -> (-31.1067, 51.9)
  line L1313 (-22.1067, 51.9) -> (-22.1067, 58.4)
  line L1314 (-31.1067, 51.9) -> (-22.1067, 51.9)
  line L1315 (-30.5067, 57.8) -> (-30.5067, 52.5)
  line L1316 (-22.7067, 57.8) -> (-30.5067, 57.8)
  line L1317 (-22.7067, 52.5) -> (-22.7067, 57.8)
  line L1318 (-40.36, 52.5) -> (-32.56, 52.5)
  line L1319 (-31.96, 58.4) -> (-40.96, 58.4)
  line L1320 (-40.96, 58.4) -> (-40.96, 51.9)
  line L1321 (-31.96, 51.9) -> (-31.96, 58.4)
  line L1322 (-40.96, 51.9) -> (-31.96, 51.9)
  line L1323 (-40.36, 57.8) -> (-40.36, 52.5)
  line L1324 (-32.56, 57.8) -> (-40.36, 57.8)
  line L1325 (-32.56, 52.5) -> (-32.56, 57.8)
  line L1326 (-50.2133, 52.5) -> (-42.4133, 52.5)
  line L1327 (-41.8133, 58.4) -> (-50.8133, 58.4)
  line L1328 (-50.8133, 58.4) -> (-50.8133, 51.9)
  line L1329 (-41.8133, 51.9) -> (-41.8133, 58.4)
  line L1330 (-50.8133, 51.9) -> (-41.8133, 51.9)
  line L1331 (-50.2133, 57.8) -> (-50.2133, 52.5)
  line L1332 (-42.4133, 57.8) -> (-50.2133, 57.8)
  line L1333 (-42.4133, 52.5) -> (-42.4133, 57.8)
  line L1334 (-60.0667, 52.5) -> (-52.2667, 52.5)
  line L1335 (-51.6667, 58.4) -> (-60.6667, 58.4)
  line L1336 (-60.6667, 58.4) -> (-60.6667, 51.9)
  line L1337 (-51.6667, 51.9) -> (-51.6667, 58.4)
  line L1338 (-60.6667, 51.9) -> (-51.6667, 51.9)
  line L1339 (-60.0667, 57.8) -> (-60.0667, 52.5)
  line L1340 (-52.2667, 57.8) -> (-60.0667, 57.8)
  line L1341 (-52.2667, 52.5) -> (-52.2667, 57.8)
  line L1342 (-69.92, 52.5) -> (-62.12, 52.5)
  line L1343 (-61.52, 58.4) -> (-70.52, 58.4)
  line L1344 (-70.52, 58.4) -> (-70.52, 51.9)
  line L1345 (-61.52, 51.9) -> (-61.52, 58.4)
  line L1346 (-70.52, 51.9) -> (-61.52, 51.9)
  line L1347 (-69.92, 57.8) -> (-69.92, 52.5)
  line L1348 (-62.12, 57.8) -> (-69.92, 57.8)
  line L1349 (-62.12, 52.5) -> (-62.12, 57.8)
  line L1350 (-79.7733, 52.5) -> (-71.9733, 52.5)
  line L1351 (-71.3733, 58.4) -> (-80.3733, 58.4)
  line L1352 (-80.3733, 58.4) -> (-80.3733, 51.9)
  line L1353 (-71.3733, 51.9) -> (-71.3733, 58.4)
  line L1354 (-80.3733, 51.9) -> (-71.3733, 51.9)
  line L1355 (-79.7733, 57.8) -> (-79.7733, 52.5)
  line L1356 (-71.9733, 57.8) -> (-79.7733, 57.8)
  line L1357 (-71.9733, 52.5) -> (-71.9733, 57.8)
  line L1358 (-89.6267, 52.5) -> (-81.8267, 52.5)
  line L1359 (-81.2267, 58.4) -> (-90.2267, 58.4)
  line L1360 (-90.2267, 58.4) -> (-90.2267, 51.9)
  line L1361 (-81.2267, 51.9) -> (-81.2267, 58.4)
  line L1362 (-90.2267, 51.9) -> (-81.2267, 51.9)
  line L1363 (-89.6267, 57.8) -> (-89.6267, 52.5)
  line L1364 (-81.8267, 57.8) -> (-89.6267, 57.8)
  line L1365 (-81.8267, 52.5) -> (-81.8267, 57.8)
  line L1366 (-99.48, 52.5) -> (-91.68, 52.5)
  line L1367 (-91.08, 58.4) -> (-100.08, 58.4)
  line L1368 (-100.08, 58.4) -> (-100.08, 51.9)
  line L1369 (-91.08, 51.9) -> (-91.08, 58.4)
  line L1370 (-100.08, 51.9) -> (-91.08, 51.9)
  line L1371 (-99.48, 57.8) -> (-99.48, 52.5)
  line L1372 (-91.68, 57.8) -> (-99.48, 57.8)
  line L1373 (-91.68, 52.5) -> (-91.68, 57.8)
  line L1374 (-109.3333, 52.5) -> (-101.5333, 52.5)
  line L1375 (-100.9333, 58.4) -> (-109.9333, 58.4)
  line L1376 (-109.9333, 58.4) -> (-109.9333, 51.9)
  line L1377 (-100.9333, 51.9) -> (-100.9333, 58.4)
  line L1378 (-109.9333, 51.9) -> (-100.9333, 51.9)
  line L1379 (-109.3333, 57.8) -> (-109.3333, 52.5)
  line L1380 (-101.5333, 57.8) -> (-109.3333, 57.8)
  line L1381 (-101.5333, 52.5) -> (-101.5333, 57.8)
  line L1382 (-119.1867, 52.5) -> (-111.3867, 52.5)
  line L1383 (-110.7867, 58.4) -> (-119.7867, 58.4)
  line L1384 (-119.7867, 58.4) -> (-119.7867, 51.9)
  line L1385 (-110.7867, 51.9) -> (-110.7867, 58.4)
  line L1386 (-119.7867, 51.9) -> (-110.7867, 51.9)
  line L1387 (-119.1867, 57.8) -> (-119.1867, 52.5)
  line L1388 (-111.3867, 57.8) -> (-119.1867, 57.8)
  line L1389 (-111.3867, 52.5) -> (-111.3867, 57.8)
  line L1390 (-129.04, 52.5) -> (-121.24, 52.5)
  line L1391 (-120.64, 58.4) -> (-129.64, 58.4)
  line L1392 (-129.64, 58.4) -> (-129.64, 51.9)
  line L1393 (-120.64, 51.9) -> (-120.64, 58.4)
  line L1394 (-129.64, 51.9) -> (-120.64, 51.9)
  line L1395 (-129.04, 57.8) -> (-129.04, 52.5)
  line L1396 (-121.24, 57.8) -> (-129.04, 57.8)
  line L1397 (-121.24, 52.5) -> (-121.24, 57.8)
  line L1398 (-138.8933, 52.5) -> (-131.0933, 52.5)
  line L1399 (-130.4933, 58.4) -> (-139.4933, 58.4)
  line L1400 (-139.4933, 58.4) -> (-139.4933, 51.9)
  line L1401 (-130.4933, 51.9) -> (-130.4933, 58.4)
  line L1402 (-139.4933, 51.9) -> (-130.4933, 51.9)
  line L1403 (-138.8933, 57.8) -> (-138.8933, 52.5)
  line L1404 (-131.0933, 57.8) -> (-138.8933, 57.8)
  line L1405 (-131.0933, 52.5) -> (-131.0933, 57.8)
  line L1406 (-148.7467, 52.5) -> (-140.9467, 52.5)
  line L1407 (-140.3467, 58.4) -> (-149.3467, 58.4)
  line L1408 (-149.3467, 58.4) -> (-149.3467, 51.9)
  line L1409 (-140.3467, 51.9) -> (-140.3467, 58.4)
  line L1410 (-149.3467, 51.9) -> (-140.3467, 51.9)
  line L1411 (-148.7467, 57.8) -> (-148.7467, 52.5)
  line L1412 (-140.9467, 57.8) -> (-148.7467, 57.8)
  line L1413 (-140.9467, 52.5) -> (-140.9467, 57.8)
  line L1414 (-158.6, 52.5) -> (-150.8, 52.5)
  line L1415 (-150.2, 58.4) -> (-159.2, 58.4)
  line L1416 (-159.2, 58.4) -> (-159.2, 51.9)
  line L1417 (-150.2, 51.9) -> (-150.2, 58.4)
  line L1418 (-159.2, 51.9) -> (-150.2, 51.9)
  line L1419 (-158.6, 57.8) -> (-158.6, 52.5)
  line L1420 (-150.8, 57.8) -> (-158.6, 57.8)
  line L1421 (-150.8, 52.5) -> (-150.8, 57.8)
  line L1422 (-10.8, 42.48) -> (-3, 42.48)
  line L1423 (-2.4, 48.38) -> (-11.4, 48.38)
  line L1424 (-11.4, 48.38) -> (-11.4, 41.88)
  line L1425 (-2.4, 41.88) -> (-2.4, 48.38)
  line L1426 (-11.4, 41.88) -> (-2.4, 41.88)
  line L1427 (-10.8, 47.78) -> (-10.8, 42.48)
  line L1428 (-3, 47.78) -> (-10.8, 47.78)
  line L1429 (-3, 42.48) -> (-3, 47.78)
  line L1430 (-20.6533, 42.48) -> (-12.8533, 42.48)
  line L1431 (-12.2533, 48.38) -> (-21.2533, 48.38)
  line L1432 (-21.2533, 48.38) -> (-21.2533, 41.88)
  line L1433 (-12.2533, 41.88) -> (-12.2533, 48.38)
  line L1434 (-21.2533, 41.88) -> (-12.2533, 41.88)
  line L1435 (-20.6533, 47.78) -> (-20.6533, 42.48)
  line L1436 (-12.8533, 47.78) -> (-20.6533, 47.78)
  line L1437 (-12.8533, 42.48) -> (-12.8533, 47.78)
  line L1438 (-30.5067, 42.48) -> (-22.7067, 42.48)
  line L1439 (-22.1067, 48.38) -> (-31.1067, 48.38)
  line L1440 (-31.1067, 48.38) -> (-31.1067, 41.88)
  line L1441 (-22.1067, 41.88) -> (-22.1067, 48.38)
  line L1442 (-31.1067, 41.88) -> (-22.1067, 41.88)
  line L1443 (-30.5067, 47.78) -> (-30.5067, 42.48)
  line L1444 (-22.7067, 47.78) -> (-30.5067, 47.78)
  line L1445 (-22.7067, 42.48) -> (-22.7067, 47.78)
  line L1446 (-40.36, 42.48) -> (-32.56, 42.48)
  line L1447 (-31.96, 48.38) -> (-40.96, 48.38)
  line L1448 (-40.96, 48.38) -> (-40.96, 41.88)
  line L1449 (-31.96, 41.88) -> (-31.96, 48.38)
  line L1450 (-40.96, 41.88) -> (-31.96, 41.88)
  line L1451 (-40.36, 47.78) -> (-40.36, 42.48)
  line L1452 (-32.56, 47.78) -> (-40.36, 47.78)
  line L1453 (-32.56, 42.48) -> (-32.56, 47.78)
  line L1454 (-50.2133, 42.48) -> (-42.4133, 42.48)
  line L1455 (-41.8133, 48.38) -> (-50.8133, 48.38)
  line L1456 (-50.8133, 48.38) -> (-50.8133, 41.88)
  line L1457 (-41.8133, 41.88) -> (-41.8133, 48.38)
  line L1458 (-50.8133, 41.88) -> (-41.8133, 41.88)
  line L1459 (-50.2133, 47.78) -> (-50.2133, 42.48)
  line L1460 (-42.4133, 47.78) -> (-50.2133, 47.78)
  line L1461 (-42.4133, 42.48) -> (-42.4133, 47.78)
  line L1462 (-60.0667, 42.48) -> (-52.2667, 42.48)
  line L1463 (-51.6667, 48.38) -> (-60.6667, 48.38)
  line L1464 (-60.6667, 48.38) -> (-60.6667, 41.88)
  line L1465 (-51.6667, 41.88) -> (-51.6667, 48.38)
  line L1466 (-60.6667, 41.88) -> (-51.6667, 41.88)
  line L1467 (-60.0667, 47.78) -> (-60.0667, 42.48)
  line L1468 (-52.2667, 47.78) -> (-60.0667, 47.78)
  line L1469 (-52.2667, 42.48) -> (-52.2667, 47.78)
  line L1470 (-69.92, 42.48) -> (-62.12, 42.48)
  line L1471 (-61.52, 48.38) -> (-70.52, 48.38)
  line L1472 (-70.52, 48.38) -> (-70.52, 41.88)
  line L1473 (-61.52, 41.88) -> (-61.52, 48.38)
  line L1474 (-70.52, 41.88) -> (-61.52, 41.88)
  line L1475 (-69.92, 47.78) -> (-69.92, 42.48)
  line L1476 (-62.12, 47.78) -> (-69.92, 47.78)
  line L1477 (-62.12, 42.48) -> (-62.12, 47.78)
  line L1478 (-79.7733, 42.48) -> (-71.9733, 42.48)
  line L1479 (-71.3733, 48.38) -> (-80.3733, 48.38)
  line L1480 (-80.3733, 48.38) -> (-80.3733, 41.88)
  line L1481 (-71.3733, 41.88) -> (-71.3733, 48.38)
  line L1482 (-80.3733, 41.88) -> (-71.3733, 41.88)
  line L1483 (-79.7733, 47.78) -> (-79.7733, 42.48)
  line L1484 (-71.9733, 47.78) -> (-79.7733, 47.78)
  line L1485 (-71.9733, 42.48) -> (-71.9733, 47.78)
  line L1486 (-89.6267, 42.48) -> (-81.8267, 42.48)
  line L1487 (-81.2267, 48.38) -> (-90.2267, 48.38)
  line L1488 (-90.2267, 48.38) -> (-90.2267, 41.88)
  line L1489 (-81.2267, 41.88) -> (-81.2267, 48.38)
  line L1490 (-90.2267, 41.88) -> (-81.2267, 41.88)
  line L1491 (-89.6267, 47.78) -> (-89.6267, 42.48)
  line L1492 (-81.8267, 47.78) -> (-89.6267, 47.78)
  line L1493 (-81.8267, 42.48) -> (-81.8267, 47.78)
  line L1494 (-99.48, 42.48) -> (-91.68, 42.48)
  line L1495 (-91.08, 48.38) -> (-100.08, 48.38)
  line L1496 (-100.08, 48.38) -> (-100.08, 41.88)
  line L1497 (-91.08, 41.88) -> (-91.08, 48.38)
  line L1498 (-100.08, 41.88) -> (-91.08, 41.88)
  line L1499 (-99.48, 47.78) -> (-99.48, 42.48)
  line L1500 (-91.68, 47.78) -> (-99.48, 47.78)
  line L1501 (-91.68, 42.48) -> (-91.68, 47.78)
  line L1502 (-109.3333, 42.48) -> (-101.5333, 42.48)
  line L1503 (-100.9333, 48.38) -> (-109.9333, 48.38)
  line L1504 (-109.9333, 48.38) -> (-109.9333, 41.88)
  line L1505 (-100.9333, 41.88) -> (-100.9333, 48.38)
  line L1506 (-109.9333, 41.88) -> (-100.9333, 41.88)
  line L1507 (-109.3333, 47.78) -> (-109.3333, 42.48)
  line L1508 (-101.5333, 47.78) -> (-109.3333, 47.78)
  line L1509 (-101.5333, 42.48) -> (-101.5333, 47.78)
  line L1510 (-119.1867, 42.48) -> (-111.3867, 42.48)
  line L1511 (-110.7867, 48.38) -> (-119.7867, 48.38)
  line L1512 (-119.7867, 48.38) -> (-119.7867, 41.88)
  line L1513 (-110.7867, 41.88) -> (-110.7867, 48.38)
  line L1514 (-119.7867, 41.88) -> (-110.7867, 41.88)
  line L1515 (-119.1867, 47.78) -> (-119.1867, 42.48)
  line L1516 (-111.3867, 47.78) -> (-119.1867, 47.78)
  line L1517 (-111.3867, 42.48) -> (-111.3867, 47.78)
  line L1518 (-129.04, 42.48) -> (-121.24, 42.48)
  line L1519 (-120.64, 48.38) -> (-129.64, 48.38)
  line L1520 (-129.64, 48.38) -> (-129.64, 41.88)
  line L1521 (-120.64, 41.88) -> (-120.64, 48.38)
  line L1522 (-129.64, 41.88) -> (-120.64, 41.88)
  line L1523 (-129.04, 47.78) -> (-129.04, 42.48)
  line L1524 (-121.24, 47.78) -> (-129.04, 47.78)
  line L1525 (-121.24, 42.48) -> (-121.24, 47.78)
  line L1526 (-138.8933, 42.48) -> (-131.0933, 42.48)
  line L1527 (-130.4933, 48.38) -> (-139.4933, 48.38)
  line L1528 (-139.4933, 48.38) -> (-139.4933, 41.88)
  line L1529 (-130.4933, 41.88) -> (-130.4933, 48.38)
  line L1530 (-139.4933, 41.88) -> (-130.4933, 41.88)
  line L1531 (-138.8933, 47.78) -> (-138.8933, 42.48)
  line L1532 (-131.0933, 47.78) -> (-138.8933, 47.78)
  line L1533 (-131.0933, 42.48) -> (-131.0933, 47.78)
  line L1534 (-148.7467, 42.48) -> (-140.9467, 42.48)
  line L1535 (-140.3467, 48.38) -> (-149.3467, 48.38)
  line L1536 (-149.3467, 48.38) -> (-149.3467, 41.88)
  line L1537 (-140.3467, 41.88) -> (-140.3467, 48.38)
  line L1538 (-149.3467, 41.88) -> (-140.3467, 41.88)
  line L1539 (-148.7467, 47.78) -> (-148.7467, 42.48)
  line L1540 (-140.9467, 47.78) -> (-148.7467, 47.78)
  line L1541 (-140.9467, 42.48) -> (-140.9467, 47.78)
  line L1542 (-158.6, 42.48) -> (-150.8, 42.48)
  line L1543 (-150.2, 48.38) -> (-159.2, 48.38)
  line L1544 (-159.2, 48.38) -> (-159.2, 41.88)
  line L1545 (-150.2, 41.88) -> (-150.2, 48.38)
  line L1546 (-159.2, 41.88) -> (-150.2, 41.88)
  line L1547 (-158.6, 47.78) -> (-158.6, 42.48)
  line L1548 (-150.8, 47.78) -> (-158.6, 47.78)
  line L1549 (-150.8, 42.48) -> (-150.8, 47.78)
  line L1550 (-10.8, 32.46) -> (-3, 32.46)
  line L1551 (-2.4, 38.36) -> (-11.4, 38.36)
  line L1552 (-11.4, 38.36) -> (-11.4, 31.86)
  line L1553 (-2.4, 31.86) -> (-2.4, 38.36)
  line L1554 (-11.4, 31.86) -> (-2.4, 31.86)
  line L1555 (-10.8, 37.76) -> (-10.8, 32.46)
  line L1556 (-3, 37.76) -> (-10.8, 37.76)
  line L1557 (-3, 32.46) -> (-3, 37.76)
  line L1558 (-20.6533, 32.46) -> (-12.8533, 32.46)
  line L1559 (-12.2533, 38.36) -> (-21.2533, 38.36)
  line L1560 (-21.2533, 38.36) -> (-21.2533, 31.86)
  line L1561 (-12.2533, 31.86) -> (-12.2533, 38.36)
  line L1562 (-21.2533, 31.86) -> (-12.2533, 31.86)
  line L1563 (-20.6533, 37.76) -> (-20.6533, 32.46)
  line L1564 (-12.8533, 37.76) -> (-20.6533, 37.76)
  line L1565 (-12.8533, 32.46) -> (-12.8533, 37.76)
  line L1566 (-30.5067, 32.46) -> (-22.7067, 32.46)
  line L1567 (-22.1067, 38.36) -> (-31.1067, 38.36)
  line L1568 (-31.1067, 38.36) -> (-31.1067, 31.86)
  line L1569 (-22.1067, 31.86) -> (-22.1067, 38.36)
  line L1570 (-31.1067, 31.86) -> (-22.1067, 31.86)
  line L1571 (-30.5067, 37.76) -> (-30.5067, 32.46)
  line L1572 (-22.7067, 37.76) -> (-30.5067, 37.76)
  line L1573 (-22.7067, 32.46) -> (-22.7067, 37.76)
  line L1574 (-40.36, 32.46) -> (-32.56, 32.46)
  line L1575 (-31.96, 38.36) -> (-40.96, 38.36)
  line L1576 (-40.96, 38.36) -> (-40.96, 31.86)
  line L1577 (-31.96, 31.86) -> (-31.96, 38.36)
  line L1578 (-40.96, 31.86) -> (-31.96, 31.86)
  line L1579 (-40.36, 37.76) -> (-40.36, 32.46)
  line L1580 (-32.56, 37.76) -> (-40.36, 37.76)
  line L1581 (-32.56, 32.46) -> (-32.56, 37.76)
  line L1582 (-50.2133, 32.46) -> (-42.4133, 32.46)
  line L1583 (-41.8133, 38.36) -> (-50.8133, 38.36)
  line L1584 (-50.8133, 38.36) -> (-50.8133, 31.86)
  line L1585 (-41.8133, 31.86) -> (-41.8133, 38.36)
  line L1586 (-50.8133, 31.86) -> (-41.8133, 31.86)
  line L1587 (-50.2133, 37.76) -> (-50.2133, 32.46)
  line L1588 (-42.4133, 37.76) -> (-50.2133, 37.76)
  line L1589 (-42.4133, 32.46) -> (-42.4133, 37.76)
  line L1590 (-60.0667, 32.46) -> (-52.2667, 32.46)
  line L1591 (-51.6667, 38.36) -> (-60.6667, 38.36)
  line L1592 (-60.6667, 38.36) -> (-60.6667, 31.86)
  line L1593 (-51.6667, 31.86) -> (-51.6667, 38.36)
  line L1594 (-60.6667, 31.86) -> (-51.6667, 31.86)
  line L1595 (-60.0667, 37.76) -> (-60.0667, 32.46)
  line L1596 (-52.2667, 37.76) -> (-60.0667, 37.76)
  line L1597 (-52.2667, 32.46) -> (-52.2667, 37.76)
  line L1598 (-69.92, 32.46) -> (-62.12, 32.46)
  line L1599 (-61.52, 38.36) -> (-70.52, 38.36)
  line L1600 (-70.52, 38.36) -> (-70.52, 31.86)
  line L1601 (-61.52, 31.86) -> (-61.52, 38.36)
  line L1602 (-70.52, 31.86) -> (-61.52, 31.86)
  line L1603 (-69.92, 37.76) -> (-69.92, 32.46)
  line L1604 (-62.12, 37.76) -> (-69.92, 37.76)
  line L1605 (-62.12, 32.46) -> (-62.12, 37.76)
  line L1606 (-79.7733, 32.46) -> (-71.9733, 32.46)
  line L1607 (-71.3733, 38.36) -> (-80.3733, 38.36)
  line L1608 (-80.3733, 38.36) -> (-80.3733, 31.86)
  line L1609 (-71.3733, 31.86) -> (-71.3733, 38.36)
  line L1610 (-80.3733, 31.86) -> (-71.3733, 31.86)
  line L1611 (-79.7733, 37.76) -> (-79.7733, 32.46)
  line L1612 (-71.9733, 37.76) -> (-79.7733, 37.76)
  line L1613 (-71.9733, 32.46) -> (-71.9733, 37.76)
  line L1614 (-89.6267, 32.46) -> (-81.8267, 32.46)
  line L1615 (-81.2267, 38.36) -> (-90.2267, 38.36)
  line L1616 (-90.2267, 38.36) -> (-90.2267, 31.86)
  line L1617 (-81.2267, 31.86) -> (-81.2267, 38.36)
  line L1618 (-90.2267, 31.86) -> (-81.2267, 31.86)
  line L1619 (-89.6267, 37.76) -> (-89.6267, 32.46)
  line L1620 (-81.8267, 37.76) -> (-89.6267, 37.76)
  line L1621 (-81.8267, 32.46) -> (-81.8267, 37.76)
  line L1622 (-99.48, 32.46) -> (-91.68, 32.46)
  line L1623 (-91.08, 38.36) -> (-100.08, 38.36)
  line L1624 (-100.08, 38.36) -> (-100.08, 31.86)
  line L1625 (-91.08, 31.86) -> (-91.08, 38.36)
  line L1626 (-100.08, 31.86) -> (-91.08, 31.86)
  line L1627 (-99.48, 37.76) -> (-99.48, 32.46)
  line L1628 (-91.68, 37.76) -> (-99.48, 37.76)
  line L1629 (-91.68, 32.46) -> (-91.68, 37.76)
  line L1630 (-109.3333, 32.46) -> (-101.5333, 32.46)
  line L1631 (-100.9333, 38.36) -> (-109.9333, 38.36)
  line L1632 (-109.9333, 38.36) -> (-109.9333, 31.86)
  line L1633 (-100.9333, 31.86) -> (-100.9333, 38.36)